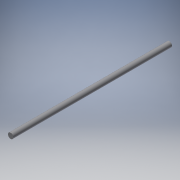
# Autodesk Inventor part: Barra
Saved by Autodesk Inventor 2019 (Build 230136000, 136)
## iProperties
Created: 2020-01-19
Part Number: Barra
Material: Generic
Document SubType Name: Modeling
Designer: peter
Density: 15.5109 g/cm^3
Appearance: Default
Mass: 23 g
Surface Area: 15.0796 cm^2
Volume: 1.48283 cm^3
Author: peter
Autodesk Inventor part; units mm, degrees
ref_plane "YZ Plane" through (0, 0, 0) normal (1, 0, 0) x (0, 1, 0)
ref_plane "XZ Plane" through (0, 0, 0) normal (0, 1, 0) x (-1, 0, 0)
ref_plane "XY Plane" through (0, 0, 0) normal (0, 0, 1) x (1, 0, 0)
sketch "Sketch1" plane through (0, 0, 0) normal (0, 0, 1) x (1, 0, 0)
  circle A0 centre (-3.4104, 4.9757) radius 2
  point P0 (0, 0)
  dimension "d1" = 4
  dimension "d1" = 4
  constraints: 1 centre point
  measures "d1" diameter of A0
extrude "Extrusion1" add sketch "Sketch1" along normal blind 118
body "Solid1"
